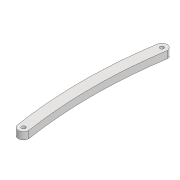
# Autodesk Inventor part: Part_4
Saved by Autodesk Inventor 2022 (Build 260153000, 153)
## iProperties
Created: 2022-04-22
Part Number: Part_4
Material: Generic
Document SubType Name: Modeling
Designer: dell
Density: 1 g/cm^3
Appearance: Default
Mass: 2.14429 g
Surface Area: 18.9003 cm^2
Volume: 2.14429 cm^3
Author: dell
Autodesk Inventor part; units mm, degrees
ref_plane "YZ Plane" through (0, 0, 0) normal (1, 0, 0) x (0, 1, 0)
ref_plane "XZ Plane" through (0, 0, 0) normal (0, 1, 0) x (-1, 0, 0)
ref_plane "XY Plane" through (0, 0, 0) normal (0, 0, 1) x (1, 0, 0)
sketch "Sketch1" plane through (0, 0, 0) normal (0, 1, 0) x (-1, 0, 0)
  line L0 (0, 0) -> (0, -77.772) construction
  line L1 (3, 0) -> (3, -77.772)
  line L2 (-3, -77.772) -> (-3, 0)
  arc A0 (3, 0) -> (-3, 0) centre (0, 0) ccw
  arc A1 (-3, -77.772) -> (3, -77.772) centre (0, -77.772) ccw
  circle A2 centre (0, 0) radius 1.1
  circle A3 centre (0, -77.772) radius 1.1
  arc A4 (-3, -77.772) -> (-3, 0) centre (-249.9572, -38.886) ccw
  arc A5 (3, -77.772) -> (3, 0) centre (-243.9572, -38.886) ccw
  point P0 (0, -38.886)
  dimension "d0" = 2.2
  dimension "d1" = 2.2
  dimension "d2" = 6
  dimension "d3" = 77.772
  dimension "d12" = 250
  dimension "d13" = 250
  constraints: 8 end point, 8 point on circle, 6 centre point, 4 tangent, 2 coincident, 1 midpoint, 1 parallel, 1 vertical
  measures "d0" diameter of A2
  measures "d1" diameter of A3
  measures "d2" distance between parallel lines of L2 L1
  measures "d3" distance of L0.end L0.start
  measures "d12" radius of A5
  measures "d13" radius of A4
extrude "Extrusion1" add sketch "Sketch1" along normal blind 4 contours A5 L1 | L1 A1 A4 A0
body "Solid1"
